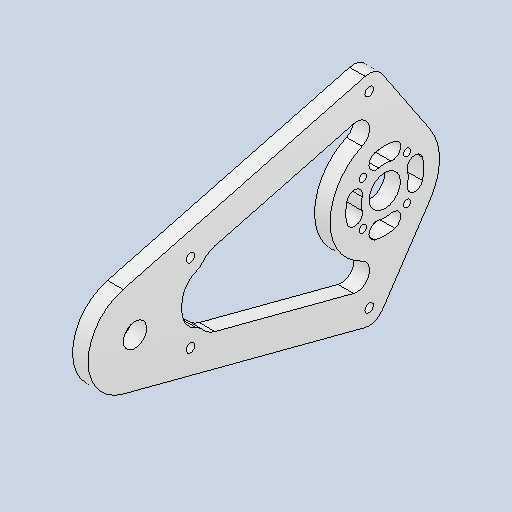
# Autodesk Inventor part: Frame (Motor Side)
Saved by Autodesk Inventor 2023 (Build 270158000, 158)
## iProperties
Created: 2022-05-22
Part Number: Frame (Motor Side)
Material: Aluminum 6061
Document SubType Name: Modeling
Designer: Nathan Cai
Density: 2.7 g/cm^3
Appearance: Aluminum - Flat
Mass: 86.2633 g
Surface Area: 157.268 cm^2
Volume: 31.9494 cm^3
Author: Nathan Cai
Autodesk Inventor part; units mm, degrees
ref_plane "YZ Plane" through (0, 0, 0) normal (1, 0, 0) x (0, 1, 0)
ref_plane "XZ Plane" through (0, 0, 0) normal (0, 1, 0) x (-1, 0, 0)
ref_plane "XY Plane" through (0, 0, 0) normal (0, 0, 1) x (1, 0, 0)
sketch "Sketch1" plane through (0, 0, 0) normal (1, 0, 0) x (0, 1, 0)
  circle A0 centre (0, 0) radius 6.35
  circle A1 centre (0, 0) radius 22.225
  line L0 (0, 0) -> (0, 101.6) construction
  circle A2 centre (0, 101.6) radius 4.7625
  circle A3 centre (0, 101.6) radius 76.2 construction
  circle A4 centre (0, 101.6) radius 19.05
  line L1 (0, 6.35) -> (38.1, 6.35) construction
  circle A5 centre (38.1, 6.35) radius 1.7526
  arc A6 (31.9576, 4.7397) -> (34.574, 11.6311) centre (38.1, 6.35) ccw
  line L2 (41.626, 1.0689) -> (12.341, -18.4838)
  line L3 (18.4273, 106.4309) -> (44.2424, 7.9603)
  line L4 (10.6971, 85.8369) -> (31.9576, 4.7397)
  line L5 (34.574, 11.6311) -> (21.9892, 3.2286) construction
  circle A7 centre (-38.1, 6.35) radius 1.7526
  arc A8 (-34.574, 11.6311) -> (-31.9576, 4.7397) centre (-38.1, 6.35) ccw
  line L6 (-41.626, 1.0689) -> (-12.341, -18.4838)
  line L7 (-18.4273, 106.4309) -> (-44.2424, 7.9603)
  line L8 (-10.6971, 85.8369) -> (-31.9576, 4.7397)
  line L9 (-34.574, 11.6311) -> (-21.9892, 3.2286)
  line L10 (0, 0) -> (0, -9.5) construction
  line L11 (0, 0) -> (9.5, 0) construction
  line L12 (0, 0) -> (-8, 0) construction
  line L13 (0, 0) -> (-12.5, 0) construction
  line L14 (0, 0) -> (-4.3437, -11.9341) construction
  line L15 (0, 0) -> (12.7, 0) construction
  line L16 (0, 0) -> (4.3437, -11.9341) construction
  line L17 (38.1, 6.35) -> (15.8856, 91.0857) construction
  circle A9 centre (19.05, 79.0153) radius 1.7526
  circle A10 centre (-19.05, 79.0153) radius 1.7526
  line L18 (-9, 9) -> (9, 9) construction
  line L19 (9, 9) -> (9, -9) construction
  line L20 (9, -9) -> (-9, -9) construction
  line L21 (-9, -9) -> (-9, 9) construction
  line L22 (-9, 9) -> (9, -9) construction
  line L23 (9, 9) -> (-9, -9) construction
  line L24 (-9, 9) -> (9, 9) construction
  circle A11 centre (9, -9) radius 1.5
  circle A12 centre (9, 9) radius 1.5
  circle A13 centre (-9, 9) radius 1.5
  circle A14 centre (-9, -9) radius 1.5
  arc A15 (3.287, 12.2673) -> (-3.287, 12.2673) centre (0, 0) ccw construction
  arc A16 (4.1088, 15.3341) -> (-4.1088, 15.3341) centre (0, 0) ccw
  arc A17 (2.4653, 9.2004) -> (-2.4653, 9.2004) centre (0, 0) ccw
  arc A18 (2.4653, 9.2004) -> (4.1088, 15.3341) centre (3.287, 12.2673) ccw
  arc A19 (-4.1088, 15.3341) -> (-2.4653, 9.2004) centre (-3.287, 12.2673) ccw
  line L25 (0, 0) -> (-3.287, 12.2673) construction
  line L26 (0, 0) -> (3.287, 12.2673) construction
  arc A20 (-9.2004, 2.4653) -> (-9.2004, -2.4653) centre (0, 0) ccw
  arc A21 (-9.2004, 2.4653) -> (-15.3341, 4.1088) centre (-12.2673, 3.287) ccw
  arc A22 (-15.3341, -4.1088) -> (-9.2004, -2.4653) centre (-12.2673, -3.287) ccw
  arc A23 (-12.2673, 3.287) -> (-12.2673, -3.287) centre (0, 0) ccw construction
  arc A24 (-15.3341, 4.1088) -> (-15.3341, -4.1088) centre (0, 0) ccw
  arc A25 (-2.4653, -9.2004) -> (2.4653, -9.2004) centre (0, 0) ccw
  arc A26 (-2.4653, -9.2004) -> (-4.1088, -15.3341) centre (-3.287, -12.2673) ccw
  arc A27 (4.1088, -15.3341) -> (2.4653, -9.2004) centre (3.287, -12.2673) ccw
  arc A28 (-3.287, -12.2673) -> (3.287, -12.2673) centre (0, 0) ccw construction
  arc A29 (-4.1088, -15.3341) -> (4.1088, -15.3341) centre (0, 0) ccw
  arc A30 (9.2004, -2.4653) -> (9.2004, 2.4653) centre (0, 0) ccw
  arc A31 (9.2004, -2.4653) -> (15.3341, -4.1088) centre (12.2673, -3.287) ccw
  arc A32 (15.3341, 4.1088) -> (9.2004, 2.4653) centre (12.2673, 3.287) ccw
  arc A33 (12.2673, -3.287) -> (12.2673, 3.287) centre (0, 0) ccw construction
  arc A34 (15.3341, -4.1088) -> (15.3341, 4.1088) centre (0, 0) ccw
  arc A35 (20.2201, 9.2249) -> (29.8796, 12.6659) centre (24.9019, 11.3609) ccw
  arc A36 (-29.8796, 12.6659) -> (-20.2201, 9.2249) centre (-24.9019, 11.3609) ccw
  line L27 (19.05, 79.0153) -> (-19.05, 79.0153) construction
  circle A37 centre (15.875, 79.0153) radius 6.35
  circle A38 centre (15.875, 79.0153) radius 1.7526
  circle A39 centre (-15.875, 79.0153) radius 6.35
  circle A40 centre (-15.875, 79.0153) radius 1.7526
  point P0 (-18.4273, 106.4309)
  point P1 (-12.341, -18.4838)
  point P2 (30.8098, 9.1178)
  point P3 (-21.9892, 3.2286)
  point P4 (-30.8098, 9.1178)
  point P5 (-20.2201, 9.2249)
  point P6 (-29.8796, 12.6659)
  point P7 (11.3244, 83.4441)
  point P8 (14.0824, 72.9236)
  point P9 (-14.0824, 72.9236)
  point P10 (-11.3244, 83.4441)
  dimension "d0" = 12.7
  dimension "d1" = 44.45
  dimension "d2" = 101.6
  dimension "d3" = 9.525
  dimension "d4" = 152.4
  dimension "d5" = 38.1
  dimension "d6" = 38.1
  dimension "d7" = 3.5052
  dimension "d8" = 12.7
  dimension "d9" = 6.35
  dimension "d10" = 12.7
  dimension "d11" = 12.7
  dimension "d15" = 9.5
  dimension "d16" = 270
  dimension "d18" = 8
  dimension "d20" = 12.5
  dimension "d35" = 70
  dimension "d36" = 3.5052
  dimension "d37" = 19.05
  dimension "d38" = 18
  dimension "d40" = 18
  dimension "d41" = 3
  dimension "d44" = 360
  dimension "d46" = 12.7
  dimension "d47" = 30
  dimension "d48" = 6.35
  dimension "d49" = 75
  dimension "d52" = 360
  dimension "d54" = 12.7
  dimension "d55" = 3.5052
  dimension "d56" = 15.875
  constraints: 58 point on circle, 56 end point, 41 centre point, 17 symmetric about line, 14 coincident, 11 tangent, 6 parallel, 5 horizontal, 4 point on line, 3 equal length, 2 midpoint, 2 perpendicular, 1 collinear, 1 vertical, 64 other
  measures "d0" diameter of A0
  measures "d1" diameter of A1
  measures "d2" distance of L0.start L0.end
  measures "d3" diameter of A2
  measures "d4" diameter of A3
  measures "d5" diameter of A4
  measures "d6" distance of L1.start L1.end
  measures "d7" diameter of A5
  measures "d8" diameter of A6
  measures "d9" distance from line of A0.centre L1
  measures "d10" distance between parallel lines of L3 L4
  measures "d11" distance between parallel lines of L2 L5
  measures "d15" distance of L0.start L10.end
  measures "d18" distance of L0.start L12.end
  measures "d20" distance of L0.start L13.end
  measures "d35" angle of L11 L16
  measures "d36" diameter of A9
  measures "d37" distance from line of L0 L27.start
  measures "d38" distance of L18.start L18.end
  measures "d40" distance of L18.end L19.end
  measures "d41" diameter of A11
  measures "d46" radius of A15
  measures "d47" angle of L26 L25
  measures "d48" diameter of A19
  measures "d49" angle of L11 L26
  measures "d54" diameter of A37
  measures "d55" diameter of A38
  measures "d56" distance from line of L0 A38.centre
extrude "Extrusion1" add sketch "Sketch1" along normal blind 6.35 contours A1 | A1 A35 L4 A6 L2 | A1 L9 A36 | L4 A37 A4 L3 A6 | L6 A8 L8 L9 A1 | L9 L8 A36 | A37 L4 | L4 A37 | A8 L9 L8 | L9 A8 L7 A4 L8 A39 | A4 | A39 L8 | L8 A39 | A9 A38 | A40 A10 picked at (19.7267, 78.8731) picked at (-19.7267, 79.1575)
fillet "Fillet1" radius 9.525 6 edges at (3.175, 10.6971, 85.8369) (3.175, -10.6971, 85.8369) (3.175, 14.0824, 72.9236) (3.175, 11.3244, 83.4441) (3.175, -11.3244, 83.4441) (3.175, -14.0824, 72.9236)
equation "\"d10\" = d8"
equation "\"d11\" = d10"
equation "\"d37\" = Leg_Offset"
equation "\"d56\" = Leg_Mounts"
equation "\"Leg_Offset\" = 19.05"
equation "\"Leg_Mounts\" = 15.875"
body "Solid1"
